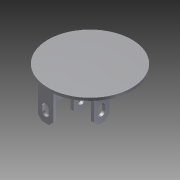
# Autodesk Inventor part: YB16SKW01
Saved by Autodesk Inventor 2015 SP1 (Build 190203100, 203)
## iProperties
Category: Electrical
Company: Autodesk Inc.
Created: 2013-12-31
Part Number: YB16SKW01
Catalog Web Link: www.cadenas.de
Description: Panel Mount Illuminated Pushbuttons_terminal-
Vendor: NKK Switches
Document SubType Name: Modeling
Designer: Autodesk Inc.
Manufacturer: NKKSWITCHES
Density: 1 g/cm^3
Material: Generic
Appearance: RGB(191.25000000000000,191.25000000000000,191.25000000000000)
Title: YB16SKW01-05-BBterminal
Author: Autodesk Inc.
Autodesk Inventor part; units mm, degrees
sketch "Sketch_1" plane through (0, 0.508, 0) normal (0, 1, 0) x (1, 0, 0)
  circle A0 centre (0, 0) radius 7.619
  constraints: 1 centre point
extrude "Extrusion1" add sketch "Sketch_1" along normal blind 0.4877
sketch "Sketch_8" plane through (1.8542, 0, 0) normal (1, 0, 0) x (0, 0, -1)
  line L0 (-1.397, -6.5532) -> (-0.635, -7.3152)
  line L1 (-0.635, -7.3152) -> (0.635, -7.3152)
  line L2 (0.635, -7.3152) -> (1.397, -6.5532)
  line L3 (1.397, -6.5532) -> (1.397, 0.762)
  line L4 (1.397, 0.762) -> (-1.397, 0.762)
  line L5 (-1.397, 0.762) -> (-1.397, -6.5532)
  line L6 (-0.5969, -4.8768) -> (-0.5969, -5.6896)
  arc A0 (-0.5969, -5.6896) -> (0.5969, -5.6896) centre (0, -5.6896) ccw
  line L7 (0.5969, -5.6896) -> (0.5969, -4.8768)
  arc A1 (0.5969, -4.8768) -> (-0.5969, -4.8768) centre (0, -4.8768) ccw
  constraints: 16 end point, 4 point on circle, 2 centre point
extrude "Extrusion2" add sketch "Sketch_8" along normal mid plane 0.508
sketch "Sketch_7" plane through (-1.8542, 0, 0) normal (1, 0, 0) x (0, 0, -1)
  line L0 (-1.397, -6.5532) -> (-0.635, -7.3152)
  line L1 (-0.635, -7.3152) -> (0.635, -7.3152)
  line L2 (0.635, -7.3152) -> (1.397, -6.5532)
  line L3 (1.397, -6.5532) -> (1.397, 0.762)
  line L4 (1.397, 0.762) -> (-1.397, 0.762)
  line L5 (-1.397, 0.762) -> (-1.397, -6.5532)
  line L6 (-0.5969, -4.8768) -> (-0.5969, -5.6896)
  arc A0 (-0.5969, -5.6896) -> (0.5969, -5.6896) centre (0, -5.6896) ccw
  line L7 (0.5969, -5.6896) -> (0.5969, -4.8768)
  arc A1 (0.5969, -4.8768) -> (-0.5969, -4.8768) centre (0, -4.8768) ccw
  constraints: 16 end point, 4 point on circle, 2 centre point
extrude "Extrusion3" add sketch "Sketch_7" along normal mid plane 0.508
sketch "Sketch_9" plane through (-5.5499, 0, 0) normal (1, 0, 0) x (0, 0, -1)
  line L0 (-1.397, -6.5532) -> (-0.635, -7.3152)
  line L1 (-0.635, -7.3152) -> (0.635, -7.3152)
  line L2 (0.635, -7.3152) -> (1.397, -6.5532)
  line L3 (1.397, -6.5532) -> (1.397, 0.762)
  line L4 (1.397, 0.762) -> (-1.397, 0.762)
  line L5 (-1.397, 0.762) -> (-1.397, -6.5532)
  line L6 (-0.5969, -4.8768) -> (-0.5969, -5.6896)
  arc A0 (-0.5969, -5.6896) -> (0.5969, -5.6896) centre (0, -5.6896) ccw
  line L7 (0.5969, -5.6896) -> (0.5969, -4.8768)
  arc A1 (0.5969, -4.8768) -> (-0.5969, -4.8768) centre (0, -4.8768) ccw
  constraints: 16 end point, 4 point on circle, 2 centre point
extrude "Extrusion4" add sketch "Sketch_9" along normal mid plane 0.508
sketch "Sketch_2" plane through (0, 0, 4.8514) normal (0, 0, 1) x (1, 0, 0)
  line L0 (-4.3942, -6.5532) -> (-3.6322, -7.3152)
  line L1 (-3.6322, -7.3152) -> (-2.3622, -7.3152)
  line L2 (-2.3622, -7.3152) -> (-1.6002, -6.5532)
  line L3 (-1.6002, -6.5532) -> (-1.6002, 0.762)
  line L4 (-1.6002, 0.762) -> (-4.3942, 0.762)
  line L5 (-4.3942, 0.762) -> (-4.3942, -6.5532)
  line L6 (-3.5941, -4.8768) -> (-3.5941, -5.6896)
  arc A0 (-3.5941, -5.6896) -> (-2.4003, -5.6896) centre (-2.9972, -5.6896) ccw
  line L7 (-2.4003, -5.6896) -> (-2.4003, -4.8768)
  arc A1 (-2.4003, -4.8768) -> (-3.5941, -4.8768) centre (-2.9972, -4.8768) ccw
  constraints: 16 end point, 4 point on circle, 2 centre point
extrude "Extrusion5" add sketch "Sketch_2" along normal mid plane 0.508
sketch "Sketch_11" plane through (0, 0, -4.8514) normal (0, 0, 1) x (1, 0, 0)
  line L0 (-4.3942, -6.5532) -> (-3.6322, -7.3152)
  line L1 (-3.6322, -7.3152) -> (-2.3622, -7.3152)
  line L2 (-2.3622, -7.3152) -> (-1.6002, -6.5532)
  line L3 (-1.6002, -6.5532) -> (-1.6002, 0.762)
  line L4 (-1.6002, 0.762) -> (-4.3942, 0.762)
  line L5 (-4.3942, 0.762) -> (-4.3942, -6.5532)
  line L6 (-3.5941, -4.8768) -> (-3.5941, -5.6896)
  arc A0 (-3.5941, -5.6896) -> (-2.4003, -5.6896) centre (-2.9972, -5.6896) ccw
  line L7 (-2.4003, -5.6896) -> (-2.4003, -4.8768)
  arc A1 (-2.4003, -4.8768) -> (-3.5941, -4.8768) centre (-2.9972, -4.8768) ccw
  constraints: 16 end point, 4 point on circle, 2 centre point
extrude "Extrusion6" add sketch "Sketch_11" along normal mid plane 0.508
ref_plane "terminal_to_body_XY" through (0, 16.9926, 0) normal (0, 1, 0) x (1, 0, 0)
ref_plane "terminal_to_body_YZ" through (0, 16.9926, 0) normal (1, 0, 0) x (0, 0, -1)
ref_plane "terminal_to_body_ZX" through (0, 16.9926, 0) normal (0, 0, -1) x (0, 1, 0)
body "Solid1"
